Autodesk Inventor part; units mm, degrees
(part 2 of 3)
  spline S285 degree 3 poles (-158.7452, 2.7796) (-159.3519, 3.3863) (-159.5334, 4.2987) (-159.205, 5.0914) knots 0 0 0 0 1 1 1 1 construction
  spline S286 degree 3 poles (-159.205, 5.0914) (-158.8767, 5.8841) (-158.1032, 6.4009) (-157.2452, 6.4009) knots 0 0 0 0 1 1 1 1 construction
  arc A68 (-155.1239, 4.2796) -> (-157.2452, 6.4009) centre (-157.2452, 4.2796) ccw construction
  spline S287 degree 3 poles (-145.4719, 23.3296) (-145.4719, 22.4716) (-145.9887, 21.6981) (-146.7814, 21.3698) knots 0 0 0 0 1 1 1 1 construction
  spline S288 degree 3 poles (-146.7814, 21.3698) (-147.5741, 21.0414) (-148.4865, 21.2229) (-149.0932, 21.8296) knots 0 0 0 0 1 1 1 1 construction
  spline S289 degree 3 poles (-149.0932, 21.8296) (-149.6999, 22.4363) (-149.8814, 23.3487) (-149.553, 24.1414) knots 0 0 0 0 1 1 1 1 construction
  spline S290 degree 3 poles (-149.553, 24.1414) (-149.2247, 24.9341) (-148.4512, 25.4509) (-147.5932, 25.4509) knots 0 0 0 0 1 1 1 1 construction
  arc A69 (-145.4719, 23.3296) -> (-147.5932, 25.4509) centre (-147.5932, 23.3296) ccw construction
  spline S291 degree 3 poles (-136.0739, 4.2796) (-136.0739, 3.4216) (-136.5907, 2.6481) (-137.3834, 2.3198) knots 0 0 0 0 1 1 1 1 construction
  spline S292 degree 3 poles (-137.3834, 2.3198) (-138.1761, 1.9914) (-139.0885, 2.1729) (-139.6952, 2.7796) knots 0 0 0 0 1 1 1 1 construction
  spline S293 degree 3 poles (-139.6952, 2.7796) (-140.3019, 3.3863) (-140.4834, 4.2987) (-140.155, 5.0914) knots 0 0 0 0 1 1 1 1 construction
  spline S294 degree 3 poles (-140.155, 5.0914) (-139.8267, 5.8841) (-139.0532, 6.4009) (-138.1952, 6.4009) knots 0 0 0 0 1 1 1 1 construction
  arc A70 (-136.0739, 4.2796) -> (-138.1952, 6.4009) centre (-138.1952, 4.2796) ccw construction
  spline S295 degree 3 poles (-140.6459, -33.8204) (-140.6459, -34.6784) (-141.1627, -35.4519) (-141.9554, -35.7802) knots 0 0 0 0 1 1 1 1 construction
  spline S296 degree 3 poles (-141.9554, -35.7802) (-142.7481, -36.1086) (-143.6605, -35.9271) (-144.2672, -35.3204) knots 0 0 0 0 1 1 1 1 construction
  spline S297 degree 3 poles (-144.2672, -35.3204) (-144.8739, -34.7137) (-145.0554, -33.8013) (-144.727, -33.0086) knots 0 0 0 0 1 1 1 1 construction
  spline S298 degree 3 poles (-144.727, -33.0086) (-144.3987, -32.2159) (-143.6252, -31.6991) (-142.7672, -31.6991) knots 0 0 0 0 1 1 1 1 construction
  arc A71 (-140.6459, -33.8204) -> (-142.7672, -31.6991) centre (-142.7672, -33.8204) ccw construction
  spline S299 degree 3 poles (-131.2479, -14.7704) (-131.2479, -15.6284) (-131.7647, -16.4019) (-132.5574, -16.7302) knots 0 0 0 0 1 1 1 1 construction
  spline S300 degree 3 poles (-132.5574, -16.7302) (-133.3501, -17.0586) (-134.2625, -16.8771) (-134.8692, -16.2704) knots 0 0 0 0 1 1 1 1 construction
  spline S301 degree 3 poles (-134.8692, -16.2704) (-135.4759, -15.6637) (-135.6574, -14.7513) (-135.329, -13.9586) knots 0 0 0 0 1 1 1 1 construction
  spline S302 degree 3 poles (-135.329, -13.9586) (-135.0007, -13.1659) (-134.2272, -12.6491) (-133.3692, -12.6491) knots 0 0 0 0 1 1 1 1 construction
  arc A72 (-131.2479, -14.7704) -> (-133.3692, -12.6491) centre (-133.3692, -14.7704) ccw construction
  spline S303 degree 3 poles (-121.5959, -33.8204) (-121.5959, -34.6784) (-122.1127, -35.4519) (-122.9054, -35.7802) knots 0 0 0 0 1 1 1 1 construction
  spline S304 degree 3 poles (-122.9054, -35.7802) (-123.6981, -36.1086) (-124.6105, -35.9271) (-125.2172, -35.3204) knots 0 0 0 0 1 1 1 1 construction
  spline S305 degree 3 poles (-125.2172, -35.3204) (-125.8239, -34.7137) (-126.0054, -33.8013) (-125.677, -33.0086) knots 0 0 0 0 1 1 1 1 construction
  spline S306 degree 3 poles (-125.677, -33.0086) (-125.3487, -32.2159) (-124.5752, -31.6991) (-123.7172, -31.6991) knots 0 0 0 0 1 1 1 1 construction
  arc A73 (-121.5959, -33.8204) -> (-123.7172, -31.6991) centre (-123.7172, -33.8204) ccw construction
  arc A74 (-102.5459, -33.8204) -> (-104.6672, -31.6991) centre (-104.6672, -33.8204) ccw construction
  spline S307 degree 3 poles (-102.5459, -33.8204) (-102.5459, -34.6784) (-103.0627, -35.4519) (-103.8554, -35.7802) knots 0 0 0 0 1 1 1 1 construction
  spline S308 degree 3 poles (-103.8554, -35.7802) (-104.6481, -36.1086) (-105.5605, -35.9271) (-106.1672, -35.3204) knots 0 0 0 0 1 1 1 1 construction
  spline S309 degree 3 poles (-106.1672, -35.3204) (-106.7739, -34.7137) (-106.9554, -33.8013) (-106.627, -33.0086) knots 0 0 0 0 1 1 1 1 construction
  spline S310 degree 3 poles (-106.627, -33.0086) (-106.2987, -32.2159) (-105.5252, -31.6991) (-104.6672, -31.6991) knots 0 0 0 0 1 1 1 1 construction
  spline S311 degree 3 poles (-112.1979, -14.7704) (-112.1979, -15.6284) (-112.7147, -16.4019) (-113.5074, -16.7302) knots 0 0 0 0 1 1 1 1 construction
  spline S312 degree 3 poles (-113.5074, -16.7302) (-114.3001, -17.0586) (-115.2125, -16.8771) (-115.8192, -16.2704) knots 0 0 0 0 1 1 1 1 construction
  spline S313 degree 3 poles (-115.8192, -16.2704) (-116.4259, -15.6637) (-116.6074, -14.7513) (-116.279, -13.9586) knots 0 0 0 0 1 1 1 1 construction
  spline S314 degree 3 poles (-116.279, -13.9586) (-115.9507, -13.1659) (-115.1772, -12.6491) (-114.3192, -12.6491) knots 0 0 0 0 1 1 1 1 construction
  arc A75 (-112.1979, -14.7704) -> (-114.3192, -12.6491) centre (-114.3192, -14.7704) ccw construction
  line L28 (-145.8754, -43.9454) -> (-139.8754, -43.9454) construction
  line L29 (-139.8754, -43.9454) -> (-139.8754, -58.9454) construction
  line L30 (-139.8754, -58.9454) -> (-145.8754, -58.9454) construction
  line L31 (-145.8754, -58.9454) -> (-145.8754, -43.9454) construction
  spline S315 degree 3 poles (-134.5894, 49.9986) (-135.3821, 49.6702) (-136.2945, 49.8517) (-136.9012, 50.4584) knots 0 0 0 0 1 1 1 1 construction
  spline S316 degree 3 poles (-136.9012, 50.4584) (-137.5079, 51.0651) (-137.6894, 51.9775) (-137.361, 52.7702) knots 0 0 0 0 1 1 1 1 construction
  spline S317 degree 3 poles (-137.361, 52.7702) (-137.0327, 53.5629) (-136.2592, 54.0797) (-135.4012, 54.0797) knots 0 0 0 0 1 1 1 1 construction
  arc A76 (-133.2799, 51.9584) -> (-135.4012, 54.0797) centre (-135.4012, 51.9584) ccw construction
  spline S318 degree 3 poles (-133.2799, 51.9584) (-133.2799, 51.1004) (-133.7967, 50.3269) (-134.5894, 49.9986) knots 0 0 0 0 1 1 1 1 construction
  spline S319 degree 3 poles (-113.0252, 50.4864) (-113.6319, 51.0931) (-113.8134, 52.0055) (-113.485, 52.7982) knots 0 0 0 0 1 1 1 1 construction
  spline S320 degree 3 poles (-113.485, 52.7982) (-113.1567, 53.5909) (-112.3832, 54.1077) (-111.5252, 54.1077) knots 0 0 0 0 1 1 1 1 construction
  arc A77 (-109.4039, 51.9864) -> (-111.5252, 54.1077) centre (-111.5252, 51.9864) ccw construction
  spline S321 degree 3 poles (-109.4039, 51.9864) (-109.4039, 51.1284) (-109.9207, 50.3549) (-110.7134, 50.0266) knots 0 0 0 0 1 1 1 1 construction
  spline S322 degree 3 poles (-110.7134, 50.0266) (-111.5061, 49.6982) (-112.4185, 49.8797) (-113.0252, 50.4864) knots 0 0 0 0 1 1 1 1 construction
  arc A78 (-108.25, 37.6384) -> (-110, 39.3884) centre (-110, 37.6384) ccw construction
  spline S323 degree 3 poles (-108.25, 37.6384) (-108.25, 36.9306) (-108.6764, 36.2925) (-109.3303, 36.0216) knots 0 0 0 0 1 1 1 1 construction
  spline S324 degree 3 poles (-109.3303, 36.0216) (-109.9842, 35.7507) (-110.7369, 35.9005) (-111.2374, 36.401) knots 0 0 0 0 1 1 1 1 construction
  spline S325 degree 3 poles (-111.2374, 36.401) (-111.7379, 36.9015) (-111.8877, 37.6542) (-111.6168, 38.3081) knots 0 0 0 0 1 1 1 1 construction
  spline S326 degree 3 poles (-111.6168, 38.3081) (-111.3459, 38.962) (-110.7078, 39.3884) (-110, 39.3884) knots 0 0 0 0 1 1 1 1 construction
  arc A79 (-117.0239, 4.2796) -> (-119.1452, 6.4009) centre (-119.1452, 4.2796) ccw construction
  spline S327 degree 3 poles (-117.0239, 4.2796) (-117.0239, 3.4216) (-117.5407, 2.6481) (-118.3334, 2.3198) knots 0 0 0 0 1 1 1 1 construction
  spline S328 degree 3 poles (-118.3334, 2.3198) (-119.1261, 1.9914) (-120.0385, 2.1729) (-120.6452, 2.7796) knots 0 0 0 0 1 1 1 1 construction
  spline S329 degree 3 poles (-120.6452, 2.7796) (-121.2519, 3.3863) (-121.4334, 4.2987) (-121.105, 5.0914) knots 0 0 0 0 1 1 1 1 construction
  spline S330 degree 3 poles (-121.105, 5.0914) (-120.7767, 5.8841) (-120.0032, 6.4009) (-119.1452, 6.4009) knots 0 0 0 0 1 1 1 1 construction
  arc A80 (-107.3719, 23.3296) -> (-109.4932, 25.4509) centre (-109.4932, 23.3296) ccw construction
  spline S331 degree 3 poles (-107.3719, 23.3296) (-107.3719, 22.4716) (-107.8887, 21.6981) (-108.6814, 21.3698) knots 0 0 0 0 1 1 1 1 construction
  spline S332 degree 3 poles (-108.6814, 21.3698) (-109.4741, 21.0414) (-110.3865, 21.2229) (-110.9932, 21.8296) knots 0 0 0 0 1 1 1 1 construction
  spline S333 degree 3 poles (-110.9932, 21.8296) (-111.5999, 22.4363) (-111.7814, 23.3487) (-111.453, 24.1414) knots 0 0 0 0 1 1 1 1 construction
  spline S334 degree 3 poles (-111.453, 24.1414) (-111.1247, 24.9341) (-110.3512, 25.4509) (-109.4932, 25.4509) knots 0 0 0 0 1 1 1 1 construction
  arc A81 (-126.4219, 23.3296) -> (-128.5432, 25.4509) centre (-128.5432, 23.3296) ccw construction
  spline S335 degree 3 poles (-126.4219, 23.3296) (-126.4219, 22.158) (-127.3716, 21.2083) (-128.5432, 21.2083) knots 0 0 0 0 1 1 1 1 construction
  spline S336 degree 3 poles (-128.5432, 21.2083) (-129.7148, 21.2083) (-130.6645, 22.158) (-130.6645, 23.3296) knots 0 0 0 0 1 1 1 1 construction
  spline S337 degree 3 poles (-130.6645, 23.3296) (-130.6645, 24.5012) (-129.7148, 25.4509) (-128.5432, 25.4509) knots 0 0 0 0 1 1 1 1 construction
  arc A82 (-97.9739, 4.2008) -> (-100.0952, 6.3221) centre (-100.0952, 4.2008) ccw construction
  spline S338 degree 3 poles (-97.9739, 4.2008) (-97.9739, 3.3428) (-98.4907, 2.5693) (-99.2834, 2.241) knots 0 0 0 0 1 1 1 1 construction
  spline S339 degree 3 poles (-99.2834, 2.241) (-100.0761, 1.9126) (-100.9885, 2.0941) (-101.5952, 2.7008) knots 0 0 0 0 1 1 1 1 construction
  spline S340 degree 3 poles (-101.5952, 2.7008) (-102.2019, 3.3075) (-102.3834, 4.2199) (-102.055, 5.0126) knots 0 0 0 0 1 1 1 1 construction
  spline S341 degree 3 poles (-102.055, 5.0126) (-101.7267, 5.8053) (-100.9532, 6.3221) (-100.0952, 6.3221) knots 0 0 0 0 1 1 1 1 construction
  spline S342 degree 3 poles (-108.25, -57.5) (-108.25, -58.2078) (-108.6764, -58.8459) (-109.3303, -59.1168) knots 0 0 0 0 1 1 1 1 construction
  spline S343 degree 3 poles (-109.3303, -59.1168) (-109.9842, -59.3877) (-110.7369, -59.2379) (-111.2374, -58.7374) knots 0 0 0 0 1 1 1 1 construction
  spline S344 degree 3 poles (-111.2374, -58.7374) (-111.7379, -58.2369) (-111.8877, -57.4842) (-111.6168, -56.8303) knots 0 0 0 0 1 1 1 1 construction
  spline S345 degree 3 poles (-111.6168, -56.8303) (-111.3459, -56.1764) (-110.7078, -55.75) (-110, -55.75) knots 0 0 0 0 1 1 1 1 construction
  arc A83 (-108.25, -57.5) -> (-110, -55.75) centre (-110, -57.5) ccw construction
  spline S346 degree 3 poles (-93.1479, -14.7704) (-93.1479, -15.6284) (-93.6647, -16.4019) (-94.4574, -16.7302) knots 0 0 0 0 1 1 1 1 construction
  spline S347 degree 3 poles (-94.4574, -16.7302) (-95.2501, -17.0586) (-96.1625, -16.8771) (-96.7692, -16.2704) knots 0 0 0 0 1 1 1 1 construction
  spline S348 degree 3 poles (-96.7692, -16.2704) (-97.3759, -15.6637) (-97.5574, -14.7513) (-97.229, -13.9586) knots 0 0 0 0 1 1 1 1 construction
  spline S349 degree 3 poles (-97.229, -13.9586) (-96.9007, -13.1659) (-96.1272, -12.6491) (-95.2692, -12.6491) knots 0 0 0 0 1 1 1 1 construction
  spline S350 degree 3 poles (-95.2692, -12.6491) (-94.0976, -12.6491) (-93.1479, -13.5988) (-93.1479, -14.7704) knots 0 0 0 0 1 1 1 1 construction
  spline S351 degree 3 poles (-83.4959, -33.8204) (-83.4959, -34.6784) (-84.0127, -35.4519) (-84.8054, -35.7802) knots 0 0 0 0 1 1 1 1 construction
  spline S352 degree 3 poles (-84.8054, -35.7802) (-85.5981, -36.1086) (-86.5105, -35.9271) (-87.1172, -35.3204) knots 0 0 0 0 1 1 1 1 construction
  spline S353 degree 3 poles (-87.1172, -35.3204) (-87.7239, -34.7137) (-87.9054, -33.8013) (-87.577, -33.0086) knots 0 0 0 0 1 1 1 1 construction
  spline S354 degree 3 poles (-87.577, -33.0086) (-87.2487, -32.2159) (-86.4752, -31.6991) (-85.6172, -31.6991) knots 0 0 0 0 1 1 1 1 construction
  spline S355 degree 3 poles (-85.6172, -31.6991) (-84.4456, -31.6991) (-83.4959, -32.6488) (-83.4959, -33.8204) knots 0 0 0 0 1 1 1 1 construction
  spline S356 degree 3 poles (-89.1492, 50.4864) (-89.7559, 51.0931) (-89.9374, 52.0055) (-89.609, 52.7982) knots 0 0 0 0 1 1 1 1 construction
  spline S357 degree 3 poles (-89.609, 52.7982) (-89.2807, 53.5909) (-88.5072, 54.1077) (-87.6492, 54.1077) knots 0 0 0 0 1 1 1 1 construction
  arc A84 (-85.5279, 51.9864) -> (-87.6492, 54.1077) centre (-87.6492, 51.9864) ccw construction
  spline S358 degree 3 poles (-85.5279, 51.9864) (-85.5279, 51.1284) (-86.0447, 50.3549) (-86.8374, 50.0266) knots 0 0 0 0 1 1 1 1 construction
  spline S359 degree 3 poles (-86.8374, 50.0266) (-87.6301, 49.6982) (-88.5425, 49.8797) (-89.1492, 50.4864) knots 0 0 0 0 1 1 1 1 construction
  spline S360 degree 3 poles (-56.6432, 50.4864) (-57.2499, 51.0931) (-57.4314, 52.0055) (-57.103, 52.7982) knots 0 0 0 0 1 1 1 1 construction
  spline S361 degree 3 poles (-57.103, 52.7982) (-56.7747, 53.5909) (-56.0012, 54.1077) (-55.1432, 54.1077) knots 0 0 0 0 1 1 1 1 construction
  arc A85 (-53.0219, 51.9864) -> (-55.1432, 54.1077) centre (-55.1432, 51.9864) ccw construction
  spline S362 degree 3 poles (-53.0219, 51.9864) (-53.0219, 51.1284) (-53.5387, 50.3549) (-54.3314, 50.0266) knots 0 0 0 0 1 1 1 1 construction
  spline S363 degree 3 poles (-54.3314, 50.0266) (-55.1241, 49.6982) (-56.0365, 49.8797) (-56.6432, 50.4864) knots 0 0 0 0 1 1 1 1 construction
  spline S364 degree 3 poles (-72.8932, 21.8296) (-73.4999, 22.4363) (-73.6814, 23.3487) (-73.353, 24.1414) knots 0 0 0 0 1 1 1 1 construction
  spline S365 degree 3 poles (-73.353, 24.1414) (-73.0247, 24.9341) (-72.2512, 25.4509) (-71.3932, 25.4509) knots 0 0 0 0 1 1 1 1 construction
  arc A86 (-69.2719, 23.3296) -> (-71.3932, 25.4509) centre (-71.3932, 23.3296) ccw construction
  spline S366 degree 3 poles (-69.2719, 23.3296) (-69.2719, 22.4716) (-69.7887, 21.6981) (-70.5814, 21.3698) knots 0 0 0 0 1 1 1 1 construction
  spline S367 degree 3 poles (-70.5814, 21.3698) (-71.3741, 21.0414) (-72.2865, 21.2229) (-72.8932, 21.8296) knots 0 0 0 0 1 1 1 1 construction
  spline S368 degree 3 poles (-53.8432, 21.8296) (-54.4499, 22.4363) (-54.6314, 23.3487) (-54.303, 24.1414) knots 0 0 0 0 1 1 1 1 construction
  spline S369 degree 3 poles (-54.303, 24.1414) (-53.9747, 24.9341) (-53.2012, 25.4509) (-52.3432, 25.4509) knots 0 0 0 0 1 1 1 1 construction
  arc A87 (-50.2219, 23.3296) -> (-52.3432, 25.4509) centre (-52.3432, 23.3296) ccw construction
  spline S370 degree 3 poles (-50.2219, 23.3296) (-50.2219, 22.4716) (-50.7387, 21.6981) (-51.5314, 21.3698) knots 0 0 0 0 1 1 1 1 construction
  spline S371 degree 3 poles (-51.5314, 21.3698) (-52.3241, 21.0414) (-53.2365, 21.2229) (-53.8432, 21.8296) knots 0 0 0 0 1 1 1 1 construction
  spline S372 degree 3 poles (-88.3219, 23.3296) (-88.3219, 22.4716) (-88.8387, 21.6981) (-89.6314, 21.3698) knots 0 0 0 0 1 1 1 1 construction
  spline S373 degree 3 poles (-89.6314, 21.3698) (-90.4241, 21.0414) (-91.3365, 21.2229) (-91.9432, 21.8296) knots 0 0 0 0 1 1 1 1 construction
  spline S374 degree 3 poles (-91.9432, 21.8296) (-92.5499, 22.4363) (-92.7314, 23.3487) (-92.403, 24.1414) knots 0 0 0 0 1 1 1 1 construction
  spline S375 degree 3 poles (-92.403, 24.1414) (-92.0747, 24.9341) (-91.3012, 25.4509) (-90.4432, 25.4509) knots 0 0 0 0 1 1 1 1 construction
  spline S376 degree 3 poles (-90.4432, 25.4509) (-89.2716, 25.4509) (-88.3219, 24.5012) (-88.3219, 23.3296) knots 0 0 0 0 1 1 1 1 construction
  spline S377 degree 3 poles (-59.129, -13.9586) (-58.8007, -13.1659) (-58.0272, -12.6491) (-57.1692, -12.6491) knots 0 0 0 0 1 1 1 1 construction
  arc A88 (-55.0479, -14.7704) -> (-57.1692, -12.6491) centre (-57.1692, -14.7704) ccw construction
  spline S378 degree 3 poles (-55.0479, -14.7704) (-55.0479, -15.6284) (-55.5647, -16.4019) (-56.3574, -16.7302) knots 0 0 0 0 1 1 1 1 construction
  spline S379 degree 3 poles (-56.3574, -16.7302) (-57.1501, -17.0586) (-58.0625, -16.8771) (-58.6692, -16.2704) knots 0 0 0 0 1 1 1 1 construction
  spline S380 degree 3 poles (-58.6692, -16.2704) (-59.2759, -15.6637) (-59.4574, -14.7513) (-59.129, -13.9586) knots 0 0 0 0 1 1 1 1 construction
  spline S381 degree 3 poles (-68.527, -33.0086) (-68.1987, -32.2159) (-67.4252, -31.6991) (-66.5672, -31.6991) knots 0 0 0 0 1 1 1 1 construction
  arc A89 (-64.4459, -33.8204) -> (-66.5672, -31.6991) centre (-66.5672, -33.8204) ccw construction
  spline S382 degree 3 poles (-64.4459, -33.8204) (-64.4459, -34.6784) (-64.9627, -35.4519) (-65.7554, -35.7802) knots 0 0 0 0 1 1 1 1 construction
  spline S383 degree 3 poles (-65.7554, -35.7802) (-66.5481, -36.1086) (-67.4605, -35.9271) (-68.0672, -35.3204) knots 0 0 0 0 1 1 1 1 construction
  spline S384 degree 3 poles (-68.0672, -35.3204) (-68.6739, -34.7137) (-68.8554, -33.8013) (-68.527, -33.0086) knots 0 0 0 0 1 1 1 1 construction
  spline S385 degree 3 poles (-78.179, -13.9586) (-77.8507, -13.1659) (-77.0772, -12.6491) (-76.2192, -12.6491) knots 0 0 0 0 1 1 1 1 construction
  arc A90 (-74.0979, -14.7704) -> (-76.2192, -12.6491) centre (-76.2192, -14.7704) ccw construction
  spline S386 degree 3 poles (-74.0979, -14.7704) (-74.0979, -15.6284) (-74.6147, -16.4019) (-75.4074, -16.7302) knots 0 0 0 0 1 1 1 1 construction
  spline S387 degree 3 poles (-75.4074, -16.7302) (-76.2001, -17.0586) (-77.1125, -16.8771) (-77.7192, -16.2704) knots 0 0 0 0 1 1 1 1 construction
  spline S388 degree 3 poles (-77.7192, -16.2704) (-78.3259, -15.6637) (-78.5074, -14.7513) (-78.179, -13.9586) knots 0 0 0 0 1 1 1 1 construction
  arc A91 (-45.3959, -33.8204) -> (-47.5172, -31.6991) centre (-47.5172, -33.8204) ccw construction
  spline S389 degree 3 poles (-45.3959, -33.8204) (-45.3959, -34.6784) (-45.9127, -35.4519) (-46.7054, -35.7802) knots 0 0 0 0 1 1 1 1 construction
  spline S390 degree 3 poles (-46.7054, -35.7802) (-47.4981, -36.1086) (-48.4105, -35.9271) (-49.0172, -35.3204) knots 0 0 0 0 1 1 1 1 construction
  spline S391 degree 3 poles (-49.0172, -35.3204) (-49.6239, -34.7137) (-49.8054, -33.8013) (-49.477, -33.0086) knots 0 0 0 0 1 1 1 1 construction
  spline S392 degree 3 poles (-49.477, -33.0086) (-49.1487, -32.2159) (-48.3752, -31.6991) (-47.5172, -31.6991) knots 0 0 0 0 1 1 1 1 construction
  arc A92 (-74.6059, -52.8704) -> (-76.7272, -50.7491) centre (-76.7272, -52.8704) ccw construction
  spline S393 degree 3 poles (-74.6059, -52.8704) (-74.6059, -53.7284) (-75.1227, -54.5019) (-75.9154, -54.8302) knots 0 0 0 0 1 1 1 1 construction
  spline S394 degree 3 poles (-75.9154, -54.8302) (-76.7081, -55.1586) (-77.6205, -54.9771) (-78.2272, -54.3704) knots 0 0 0 0 1 1 1 1 construction
  spline S395 degree 3 poles (-78.2272, -54.3704) (-78.8339, -53.7637) (-79.0154, -52.8513) (-78.687, -52.0586) knots 0 0 0 0 1 1 1 1 construction
  spline S396 degree 3 poles (-78.687, -52.0586) (-78.3587, -51.2659) (-77.5852, -50.7491) (-76.7272, -50.7491) knots 0 0 0 0 1 1 1 1 construction
  arc A93 (-59.8739, 4.2796) -> (-61.9952, 6.4009) centre (-61.9952, 4.2796) ccw construction
  spline S397 degree 3 poles (-59.8739, 4.2796) (-59.8739, 3.4216) (-60.3907, 2.6481) (-61.1834, 2.3198) knots 0 0 0 0 1 1 1 1 construction
  spline S398 degree 3 poles (-61.1834, 2.3198) (-61.9761, 1.9914) (-62.8885, 2.1729) (-63.4952, 2.7796) knots 0 0 0 0 1 1 1 1 construction
  spline S399 degree 3 poles (-63.4952, 2.7796) (-64.1019, 3.3863) (-64.2834, 4.2987) (-63.955, 5.0914) knots 0 0 0 0 1 1 1 1 construction
  spline S400 degree 3 poles (-63.955, 5.0914) (-63.6267, 5.8841) (-62.8532, 6.4009) (-61.9952, 6.4009) knots 0 0 0 0 1 1 1 1 construction
  arc A94 (-78.9239, 4.2796) -> (-81.0452, 6.4009) centre (-81.0452, 4.2796) ccw construction
  spline S401 degree 3 poles (-78.9239, 4.2796) (-78.9239, 3.4216) (-79.4407, 2.6481) (-80.2334, 2.3198) knots 0 0 0 0 1 1 1 1 construction
  spline S402 degree 3 poles (-80.2334, 2.3198) (-81.0261, 1.9914) (-81.9385, 2.1729) (-82.5452, 2.7796) knots 0 0 0 0 1 1 1 1 construction
  spline S403 degree 3 poles (-82.5452, 2.7796) (-83.1519, 3.3863) (-83.3334, 4.2987) (-83.005, 5.0914) knots 0 0 0 0 1 1 1 1 construction
  spline S404 degree 3 poles (-83.005, 5.0914) (-82.6767, 5.8841) (-81.9032, 6.4009) (-81.0452, 6.4009) knots 0 0 0 0 1 1 1 1 construction
  arc A95 (-40.8239, 4.2796) -> (-42.9452, 6.4009) centre (-42.9452, 4.2796) ccw construction
  spline S405 degree 3 poles (-40.8239, 4.2796) (-40.8239, 3.4216) (-41.3407, 2.6481) (-42.1334, 2.3198) knots 0 0 0 0 1 1 1 1 construction
  spline S406 degree 3 poles (-42.1334, 2.3198) (-42.9261, 1.9914) (-43.8385, 2.1729) (-44.4452, 2.7796) knots 0 0 0 0 1 1 1 1 construction
  spline S407 degree 3 poles (-44.4452, 2.7796) (-45.0519, 3.3863) (-45.2334, 4.2987) (-44.905, 5.0914) knots 0 0 0 0 1 1 1 1 construction
  spline S408 degree 3 poles (-44.905, 5.0914) (-44.5767, 5.8841) (-43.8032, 6.4009) (-42.9452, 6.4009) knots 0 0 0 0 1 1 1 1 construction
  spline S409 degree 3 poles (219.7443, 55.7135) (220.682, 54.7759) (221.2088, 53.5041) (221.2088, 52.178) knots 0 0 0 0 1 1 1 1 construction
  spline S410 degree 3 poles (221.2088, 52.178) (221.2088, 50.1557) (219.9906, 48.3325) (218.1222, 47.5586) knots 0 0 0 0 1 1 1 1 construction
  spline S411 degree 3 poles (218.1222, 47.5586) (216.2538, 46.7847) (214.1033, 47.2125) (212.6733, 48.6425) knots 0 0 0 0 1 1 1 1 construction
  spline S412 degree 3 poles (212.6733, 48.6425) (211.2433, 50.0725) (210.8155, 52.223) (211.5894, 54.0914) knots 0 0 0 0 1 1 1 1 construction
  spline S413 degree 3 poles (211.5894, 54.0914) (212.3633, 55.9598) (214.1865, 57.178) (216.2088, 57.178) knots 0 0 0 0 1 1 1 1 construction
  spline S414 degree 3 poles (216.2088, 57.178) (217.5349, 57.178) (218.8067, 56.6512) (219.7443, 55.7135) knots 0 0 0 0 1 1 1 1 construction
  line L32 (204.7088, -52.274) -> (219.7088, -52.274) construction
  line L33 (219.7088, -52.274) -> (219.7088, -58.274) construction
  line L34 (219.7088, -58.274) -> (204.7088, -58.274) construction
  line L35 (204.7088, -58.274) -> (204.7088, -52.274) construction
  spline S415 degree 3 poles (218.3832, 38.3081) (218.6541, 38.962) (219.2922, 39.3884) (220, 39.3884) knots 0 0 0 0 1 1 1 1 construction
  arc A96 (221.75, 37.6384) -> (220, 39.3884) centre (220, 37.6384) ccw construction
  spline S416 degree 3 poles (221.75, 37.6384) (221.75, 36.9306) (221.3236, 36.2925) (220.6697, 36.0216) knots 0 0 0 0 1 1 1 1 construction
  spline S417 degree 3 poles (220.6697, 36.0216) (220.0158, 35.7507) (219.2631, 35.9005) (218.7626, 36.401) knots 0 0 0 0 1 1 1 1 construction
  spline S418 degree 3 poles (218.7626, 36.401) (218.2621, 36.9015) (218.1123, 37.6542) (218.3832, 38.3081) knots 0 0 0 0 1 1 1 1 construction
  spline S419 degree 3 poles (146.9023, 58.0219) (147.84, 57.0843) (148.3668, 55.8125) (148.3668, 54.4864) knots 0 0 0 0 1 1 1 1 construction
  spline S420 degree 3 poles (148.3668, 54.4864) (148.3668, 52.4641) (147.1486, 50.6409) (145.2802, 49.867) knots 0 0 0 0 1 1 1 1 construction
  spline S421 degree 3 poles (145.2802, 49.867) (143.4118, 49.0931) (141.2613, 49.5209) (139.8313, 50.9509) knots 0 0 0 0 1 1 1 1 construction
  spline S422 degree 3 poles (139.8313, 50.9509) (138.4013, 52.3809) (137.9735, 54.5314) (138.7474, 56.3998) knots 0 0 0 0 1 1 1 1 construction
  spline S423 degree 3 poles (138.7474, 56.3998) (139.5213, 58.2682) (141.3445, 59.4864) (143.3668, 59.4864) knots 0 0 0 0 1 1 1 1 construction
  spline S424 degree 3 poles (143.3668, 59.4864) (144.6929, 59.4864) (145.9647, 58.9596) (146.9023, 58.0219) knots 0 0 0 0 1 1 1 1 construction
  arc A97 (111.75, 37.6384) -> (110, 39.3884) centre (110, 37.6384) ccw construction
  spline S425 degree 3 poles (111.75, 37.6384) (111.75, 36.9306) (111.3236, 36.2925) (110.6697, 36.0216) knots 0 0 0 0 1 1 1 1 construction
  spline S426 degree 3 poles (110.6697, 36.0216) (110.0158, 35.7507) (109.2631, 35.9005) (108.7626, 36.401) knots 0 0 0 0 1 1 1 1 construction
  spline S427 degree 3 poles (108.7626, 36.401) (108.2621, 36.9015) (108.1123, 37.6542) (108.3832, 38.3081) knots 0 0 0 0 1 1 1 1 construction
  spline S428 degree 3 poles (108.3832, 38.3081) (108.6541, 38.962) (109.2922, 39.3884) (110, 39.3884) knots 0 0 0 0 1 1 1 1 construction
  spline S429 degree 3 poles (47.5681, -33.8204) (47.5681, -34.6784) (47.0513, -35.4519) (46.2586, -35.7802) knots 0 0 0 0 1 1 1 1 construction
  spline S430 degree 3 poles (46.2586, -35.7802) (45.4659, -36.1086) (44.5535, -35.9271) (43.9468, -35.3204) knots 0 0 0 0 1 1 1 1 construction
  spline S431 degree 3 poles (43.9468, -35.3204) (43.3401, -34.7137) (43.1586, -33.8013) (43.487, -33.0086) knots 0 0 0 0 1 1 1 1 construction
  spline S432 degree 3 poles (43.487, -33.0086) (43.8153, -32.2159) (44.5888, -31.6991) (45.4468, -31.6991) knots 0 0 0 0 1 1 1 1 construction
  arc A98 (47.5681, -33.8204) -> (45.4468, -31.6991) centre (45.4468, -33.8204) ccw construction
  spline S433 degree 3 poles (218.3832, -23.8303) (218.6541, -23.1764) (219.2922, -22.75) (220, -22.75) knots 0 0 0 0 1 1 1 1 construction
  arc A99 (221.75, -24.5) -> (220, -22.75) centre (220, -24.5) ccw construction
  spline S434 degree 3 poles (221.75, -24.5) (221.75, -25.2078) (221.3236, -25.8459) (220.6697, -26.1168) knots 0 0 0 0 1 1 1 1 construction
  spline S435 degree 3 poles (220.6697, -26.1168) (220.0158, -26.3877) (219.2631, -26.2379) (218.7626, -25.7374) knots 0 0 0 0 1 1 1 1 construction
  spline S436 degree 3 poles (218.7626, -25.7374) (218.2621, -25.2369) (218.1123, -24.4842) (218.3832, -23.8303) knots 0 0 0 0 1 1 1 1 construction
  line L36 (204.7088, -28.274) -> (219.7088, -28.274) construction
  line L37 (219.7088, -28.274) -> (219.7088, -34.274) construction
  line L38 (219.7088, -34.274) -> (204.7088, -34.274) construction
  line L39 (204.7088, -34.274) -> (204.7088, -28.274) construction
  line L40 (151.2108, -58.772) -> (151.2108, -43.772) construction
  line L41 (151.2108, -43.772) -> (157.2108, -43.772) construction
  line L42 (157.2108, -43.772) -> (157.2108, -58.772) construction
  line L43 (157.2108, -58.772) -> (151.2108, -58.772) construction
  line L44 (175.2108, -58.772) -> (175.2108, -43.772) construction
  line L45 (175.2108, -43.772) -> (181.2108, -43.772) construction
  line L46 (181.2108, -43.772) -> (181.2108, -58.772) construction
  line L47 (181.2108, -58.772) -> (175.2108, -58.772) construction
  spline S437 degree 3 poles (191.7443, 55.7135) (192.682, 54.7759) (193.2088, 53.5041) (193.2088, 52.178) knots 0 0 0 0 1 1 1 1 construction
  spline S438 degree 3 poles (193.2088, 52.178) (193.2088, 50.1557) (191.9906, 48.3325) (190.1222, 47.5586) knots 0 0 0 0 1 1 1 1 construction
  spline S439 degree 3 poles (190.1222, 47.5586) (188.2538, 46.7847) (186.1033, 47.2125) (184.6733, 48.6425) knots 0 0 0 0 1 1 1 1 construction
  spline S440 degree 3 poles (184.6733, 48.6425) (183.2433, 50.0725) (182.8155, 52.223) (183.5894, 54.0914) knots 0 0 0 0 1 1 1 1 construction
  spline S441 degree 3 poles (183.5894, 54.0914) (184.3633, 55.9598) (186.1865, 57.178) (188.2088, 57.178) knots 0 0 0 0 1 1 1 1 construction
  spline S442 degree 3 poles (188.2088, 57.178) (189.5349, 57.178) (190.8067, 56.6512) (191.7443, 55.7135) knots 0 0 0 0 1 1 1 1 construction
  line L48 (65.6708, 3.6276) -> (50.6708, 3.6276) construction
  line L49 (50.6708, 3.6276) -> (50.6708, 9.6276) construction
  line L50 (50.6708, 9.6276) -> (65.6708, 9.6276) construction
  line L51 (65.6708, 9.6276) -> (65.6708, 3.6276) construction
  line L52 (-66.3852, 61.3884) -> (51.6148, 61.3884) construction
  line L53 (-66.3852, 42.3884) -> (-66.3852, 61.3884) construction
  line L54 (51.6148, 42.3884) -> (-66.3852, 42.3884) construction
  line L55 (-76.4012, 61.3884) -> (-76.4012, 42.3884) construction
  line L56 (-194.4012, 61.3884) -> (-76.4012, 61.3884) construction
  line L57 (-76.4012, 42.3884) -> (-194.4012, 42.3884) construction
  line L58 (-194.4012, 42.3884) -> (-194.4012, 61.3884) construction
  line L59 (-204.6412, 61.3884) -> (-204.6412, 42.3884) construction
  line L60 (-223.6412, 61.3884) -> (-204.6412, 61.3884) construction
  line L61 (-223.6412, 42.3884) -> (-223.6412, 61.3884) construction
  line L62 (-204.6412, 42.3884) -> (-223.6412, 42.3884) construction
  line L63 (71.4568, 32.8296) -> (-223.6412, 32.8296) construction
  line L64 (-223.6412, 32.8296) -> (-223.6412, -43.3204) construction
  line L65 (-223.6412, -43.3204) -> (-209.6412, -43.3204) construction
  line L66 (-209.6412, -43.3204) -> (-209.6412, -62.3704) construction
  line L67 (-209.6412, -62.3704) -> (57.4568, -62.3704) projected
  line L68 (71.4568, 32.8296) -> (-223.6412, 32.8296) construction
  line L69 (4.4528, 37.558) -> (14.2318, 37.558)
  line L70 (14.2318, 37.558) -> (14.2318, 13.9046)
  line L71 (14.2318, 13.9046) -> (4.4528, 13.9046)
  line L72 (4.4528, 13.9046) -> (4.4528, -5.3455)
  line L73 (4.4528, -5.3455) -> (9.6598, -5.3455)
  line L74 (9.6598, -5.3455) -> (9.6598, -24.1954)
  line L75 (9.6598, -24.1954) -> (0.0048, -24.1954)
  line L76 (0.0048, -24.1954) -> (0.0048, -49.2614)
  line L77 (0.0048, -49.2614) -> (8.4302, -49.2614)
  line L78 (8.4302, -49.2614) -> (8.4302, -62.3704)
  line L79 (4.6528, 61.3884) -> (4.6528, 42.3884) construction
  line L80 (4.6528, 37.758) -> (14.4318, 37.758) construction
  line L81 (14.4318, 32.8296) -> (14.4318, 13.7046) construction
  line L82 (14.4318, 13.7046) -> (4.6528, 13.7046) construction
  line L83 (4.6528, 13.7046) -> (4.6528, -5.1455) construction
  line L84 (4.6528, -5.1455) -> (9.8598, -5.1455) construction
  line L85 (9.8598, -5.1455) -> (9.8598, -24.3954) construction
  line L86 (9.8598, -24.3954) -> (0.2048, -24.3954) construction
  line L87 (0.2048, -24.3954) -> (0.2048, -49.0614) construction
  line L88 (0.2048, -49.0614) -> (8.6302, -49.0614) construction
  line L89 (8.6302, -49.0614) -> (8.6302, -62.3704) construction
  line L90 (4.4528, 61.3884) -> (4.4528, 37.558)
  circle A100 centre (-220, 37.6384) radius 3.25
  circle A101 centre (-220, -24.5) radius 3.25
  circle A102 centre (-110, 37.6384) radius 3.25
  circle A103 centre (0, 37.6384) radius 3.25
  line L91 (-223.6412, 61.3884) -> (-223.6412, -43.3204)
  line L92 (-223.6412, 61.3884) -> (4.4528, 61.3884)
  line L93 (-146.4772, -45.8679) -> (-140.4772, -45.8679)
  line L94 (-140.4772, -45.8679) -> (-140.4772, -58.2679)
  line L95 (-140.4772, -58.2679) -> (-146.4772, -58.2679)
  line L96 (-146.4772, -58.2679) -> (-146.4772, -45.8679)
  line L97 (-12.9772, -45.8679) -> (-6.9772, -45.8679)
  line L98 (-6.9772, -45.8679) -> (-6.9772, -58.2679)
  line L99 (-6.9772, -58.2679) -> (-12.9772, -58.2679)
  line L100 (-12.9772, -58.2679) -> (-12.9772, -45.8679)
  line L101 (-221.1437, 58.8909) -> (-207.1387, 58.8909)
  line L102 (-207.1387, 58.8909) -> (-207.1387, 44.8859)
  line L103 (-207.1387, 44.8859) -> (-221.1437, 44.8859)
  line L104 (-221.1437, 44.8859) -> (-221.1437, 58.8909)
  line L105 (-221.1437, 58.8909) -> (-207.1387, 44.8859) construction
  line L106 (-207.1387, 58.8909) -> (-221.1437, 44.8859) construction
  line L107 (-190.0953, 59.1041) -> (-176.0903, 59.1041)
  line L108 (-176.0903, 59.1041) -> (-176.0903, 45.0991)
  line L109 (-176.0903, 45.0991) -> (-190.0953, 45.0991)
  line L110 (-190.0953, 45.0991) -> (-190.0953, 59.1041)
  line L111 (-190.0953, 59.1041) -> (-176.0903, 45.0991) construction
  line L112 (-176.0903, 59.1041) -> (-190.0953, 45.0991) construction
  line L113 (-166.2797, 58.9889) -> (-152.2747, 58.9889)
  line L114 (-152.2747, 58.9889) -> (-152.2747, 44.9839)
  line L115 (-152.2747, 44.9839) -> (-166.2797, 44.9839)
  line L116 (-166.2797, 44.9839) -> (-166.2797, 58.9889)
  line L117 (-166.2797, 58.9889) -> (-152.2747, 44.9839) construction
  line L118 (-152.2747, 58.9889) -> (-166.2797, 44.9839) construction
  line L119 (-142.4037, 58.9609) -> (-128.3987, 58.9609)
  line L120 (-128.3987, 58.9609) -> (-128.3987, 44.9559)
  line L121 (-128.3987, 44.9559) -> (-142.4037, 44.9559)
  line L122 (-142.4037, 44.9559) -> (-142.4037, 58.9609)
  line L123 (-142.4037, 58.9609) -> (-128.3987, 44.9559) construction
  line L124 (-128.3987, 58.9609) -> (-142.4037, 44.9559) construction
  line L125 (-118.5277, 58.9889) -> (-104.5227, 58.9889)
  line L126 (-104.5227, 58.9889) -> (-104.5227, 44.9839)
  line L127 (-104.5227, 44.9839) -> (-118.5277, 44.9839)
  line L128 (-118.5277, 44.9839) -> (-118.5277, 58.9889)
  line L129 (-118.5277, 58.9889) -> (-104.5227, 44.9839) construction
  line L130 (-104.5227, 58.9889) -> (-118.5277, 44.9839) construction
  line L131 (-94.6517, 58.9889) -> (-80.6467, 58.9889)
  line L132 (-80.6467, 58.9889) -> (-80.6467, 44.9839)
  line L133 (-80.6467, 44.9839) -> (-94.6517, 44.9839)
  line L134 (-94.6517, 44.9839) -> (-94.6517, 58.9889)
  line L135 (-94.6517, 58.9889) -> (-80.6467, 44.9839) construction
  line L136 (-80.6467, 58.9889) -> (-94.6517, 44.9839) construction
  line L137 (-62.1457, 58.9889) -> (-48.1407, 58.9889)
  line L138 (-48.1407, 58.9889) -> (-48.1407, 44.9839)
  line L139 (-48.1407, 44.9839) -> (-62.1457, 44.9839)
  line L140 (-62.1457, 44.9839) -> (-62.1457, 58.9889)
  line L141 (-62.1457, 58.9889) -> (-48.1407, 44.9839) construction
  line L142 (-48.1407, 58.9889) -> (-62.1457, 44.9839) construction
  line L143 (-38.2637, 58.9889) -> (-24.2587, 58.9889)
  line L144 (-24.2587, 58.9889) -> (-24.2587, 44.9839)
  line L145 (-24.2587, 44.9839) -> (-38.2637, 44.9839)
  line L146 (-38.2637, 44.9839) -> (-38.2637, 58.9889)
  line L147 (-38.2637, 58.9889) -> (-24.2587, 44.9839) construction
  line L148 (-24.2587, 58.9889) -> (-38.2637, 44.9839) construction
  line L149 (-14.3877, 58.9889) -> (-0.3827, 58.9889)
  line L150 (-0.3827, 58.9889) -> (-0.3827, 44.9839)
  line L151 (-0.3827, 44.9839) -> (-14.3877, 44.9839)
  line L152 (-14.3877, 44.9839) -> (-14.3877, 58.9889)
  line L153 (-14.3877, 58.9889) -> (-0.3827, 44.9839) construction
  line L154 (-0.3827, 58.9889) -> (-14.3877, 44.9839) construction
  line L155 (-216.4737, 30.3321) -> (-202.4687, 30.3321)
  line L156 (-202.4687, 30.3321) -> (-202.4687, 16.3271)
  line L157 (-202.4687, 16.3271) -> (-216.4737, 16.3271)
  line L158 (-216.4737, 16.3271) -> (-216.4737, 30.3321)
  line L159 (-216.4737, 30.3321) -> (-202.4687, 16.3271) construction
  line L160 (-202.4687, 30.3321) -> (-216.4737, 16.3271) construction
  line L161 (-192.6957, 30.3321) -> (-178.6907, 30.3321)
  line L162 (-178.6907, 30.3321) -> (-178.6907, 16.3271)
  line L163 (-178.6907, 16.3271) -> (-192.6957, 16.3271)
  line L164 (-192.6957, 16.3271) -> (-192.6957, 30.3321)
  line L165 (-192.6957, 30.3321) -> (-178.6907, 16.3271) construction
  line L166 (-178.6907, 30.3321) -> (-192.6957, 16.3271) construction
  line L167 (-154.5957, 30.3321) -> (-140.5907, 30.3321)
  line L168 (-140.5907, 30.3321) -> (-140.5907, 16.3271)
  line L169 (-140.5907, 16.3271) -> (-154.5957, 16.3271)
  line L170 (-154.5957, 16.3271) -> (-154.5957, 30.3321)
  line L171 (-154.5957, 30.3321) -> (-140.5907, 16.3271) construction
  line L172 (-140.5907, 30.3321) -> (-154.5957, 16.3271) construction
  line L173 (-135.5457, 30.3321) -> (-121.5407, 30.3321)
  line L174 (-121.5407, 30.3321) -> (-121.5407, 16.3271)
  line L175 (-121.5407, 16.3271) -> (-135.5457, 16.3271)
  line L176 (-135.5457, 16.3271) -> (-135.5457, 30.3321)
  line L177 (-135.5457, 30.3321) -> (-121.5407, 16.3271) construction
  line L178 (-121.5407, 30.3321) -> (-135.5457, 16.3271) construction
  line L179 (-116.4957, 30.3321) -> (-102.4907, 30.3321)
  line L180 (-102.4907, 30.3321) -> (-102.4907, 16.3271)
  line L181 (-102.4907, 16.3271) -> (-116.4957, 16.3271)
  line L182 (-116.4957, 16.3271) -> (-116.4957, 30.3321)
  line L183 (-116.4957, 30.3321) -> (-102.4907, 16.3271) construction
  line L184 (-102.4907, 30.3321) -> (-116.4957, 16.3271) construction
  line L185 (-97.4457, 30.3321) -> (-83.4407, 30.3321)
  line L186 (-83.4407, 30.3321) -> (-83.4407, 16.3271)
  line L187 (-83.4407, 16.3271) -> (-97.4457, 16.3271)
  line L188 (-97.4457, 16.3271) -> (-97.4457, 30.3321)
  line L189 (-97.4457, 30.3321) -> (-83.4407, 16.3271) construction
  line L190 (-83.4407, 30.3321) -> (-97.4457, 16.3271) construction
  line L191 (-173.6457, 30.3321) -> (-159.6407, 30.3321)
  line L192 (-159.6407, 30.3321) -> (-159.6407, 16.3271)
  line L193 (-159.6407, 16.3271) -> (-173.6457, 16.3271)
  line L194 (-173.6457, 16.3271) -> (-173.6457, 30.3321)
  line L195 (-173.6457, 30.3321) -> (-159.6407, 16.3271) construction
  line L196 (-159.6407, 30.3321) -> (-173.6457, 16.3271) construction
  line L197 (-78.3957, 30.3321) -> (-64.3907, 30.3321)
  line L198 (-64.3907, 30.3321) -> (-64.3907, 16.3271)
  line L199 (-64.3907, 16.3271) -> (-78.3957, 16.3271)
  line L200 (-78.3957, 16.3271) -> (-78.3957, 30.3321)
  line L201 (-78.3957, 30.3321) -> (-64.3907, 16.3271) construction
  line L202 (-64.3907, 30.3321) -> (-78.3957, 16.3271) construction
  line L203 (-59.3457, 30.3321) -> (-45.3407, 30.3321)
  line L204 (-45.3407, 30.3321) -> (-45.3407, 16.3271)
  line L205 (-45.3407, 16.3271) -> (-59.3457, 16.3271)
  line L206 (-59.3457, 16.3271) -> (-59.3457, 30.3321)
  line L207 (-59.3457, 30.3321) -> (-45.3407, 16.3271) construction
  line L208 (-45.3407, 30.3321) -> (-59.3457, 16.3271) construction
  line L209 (-40.2957, 30.3321) -> (-26.2907, 30.3321)
  line L210 (-26.2907, 30.3321) -> (-26.2907, 16.3271)
  line L211 (-26.2907, 16.3271) -> (-40.2957, 16.3271)
  line L212 (-40.2957, 16.3271) -> (-40.2957, 30.3321)
  line L213 (-40.2957, 30.3321) -> (-26.2907, 16.3271) construction
  line L214 (-26.2907, 30.3321) -> (-40.2957, 16.3271) construction
  line L215 (-21.2457, 30.3321) -> (-7.2407, 30.3321)
  line L216 (-7.2407, 30.3321) -> (-7.2407, 16.3271)
  line L217 (-7.2407, 16.3271) -> (-21.2457, 16.3271)
  line L218 (-21.2457, 16.3271) -> (-21.2457, 30.3321)
  line L219 (-21.2457, 30.3321) -> (-7.2407, 16.3271) construction
  line L220 (-7.2407, 30.3321) -> (-21.2457, 16.3271) construction
  line L221 (-2.1957, 30.3321) -> (11.8093, 30.3321)
  line L222 (11.8093, 30.3321) -> (11.8093, 16.3271)
  line L223 (11.8093, 16.3271) -> (-2.1957, 16.3271)
  line L224 (-2.1957, 16.3271) -> (-2.1957, 30.3321)
  line L225 (-2.1957, 30.3321) -> (11.8093, 16.3271) construction
  line L226 (11.8093, 30.3321) -> (-2.1957, 16.3271) construction
  line L227 (-11.8477, 11.2821) -> (2.1573, 11.2821)
  line L228 (2.1573, 11.2821) -> (2.1573, -2.7229)
  line L229 (2.1573, -2.7229) -> (-11.8477, -2.7229)
  line L230 (-11.8477, -2.7229) -> (-11.8477, 11.2821)
  line L231 (-11.8477, 11.2821) -> (2.1573, -2.7229) construction
  line L232 (2.1573, 11.2821) -> (-11.8477, -2.7229) construction
  line L233 (-30.8977, 11.2821) -> (-16.8927, 11.2821)
  line L234 (-16.8927, 11.2821) -> (-16.8927, -2.7229)
  line L235 (-16.8927, -2.7229) -> (-30.8977, -2.7229)
  line L236 (-30.8977, -2.7229) -> (-30.8977, 11.2821)
  line L237 (-30.8977, 11.2821) -> (-16.8927, -2.7229) construction
  line L238 (-16.8927, 11.2821) -> (-30.8977, -2.7229) construction
  line L239 (-49.9477, 11.2821) -> (-35.9427, 11.2821)
  line L240 (-35.9427, 11.2821) -> (-35.9427, -2.7229)
  line L241 (-35.9427, -2.7229) -> (-49.9477, -2.7229)
  line L242 (-49.9477, -2.7229) -> (-49.9477, 11.2821)
  line L243 (-49.9477, 11.2821) -> (-35.9427, -2.7229) construction
  line L244 (-35.9427, 11.2821) -> (-49.9477, -2.7229) construction
  line L245 (-68.9977, 11.2821) -> (-54.9927, 11.2821)
  line L246 (-54.9927, 11.2821) -> (-54.9927, -2.7229)
  line L247 (-54.9927, -2.7229) -> (-68.9977, -2.7229)
  line L248 (-68.9977, -2.7229) -> (-68.9977, 11.2821)
  line L249 (-68.9977, 11.2821) -> (-54.9927, -2.7229) construction
  line L250 (-54.9927, 11.2821) -> (-68.9977, -2.7229) construction
  line L251 (-88.0477, 11.2821) -> (-74.0427, 11.2821)
  line L252 (-74.0427, 11.2821) -> (-74.0427, -2.7229)
  line L253 (-74.0427, -2.7229) -> (-88.0477, -2.7229)
  line L254 (-88.0477, -2.7229) -> (-88.0477, 11.2821)
  line L255 (-88.0477, 11.2821) -> (-74.0427, -2.7229) construction
  line L256 (-74.0427, 11.2821) -> (-88.0477, -2.7229) construction
  line L257 (-107.0977, 11.2033) -> (-93.0927, 11.2033)
  line L258 (-93.0927, 11.2033) -> (-93.0927, -2.8017)
  line L259 (-93.0927, -2.8017) -> (-107.0977, -2.8017)
  line L260 (-107.0977, -2.8017) -> (-107.0977, 11.2033)
  line L261 (-107.0977, 11.2033) -> (-93.0927, -2.8017) construction
  line L262 (-93.0927, 11.2033) -> (-107.0977, -2.8017) construction
  line L263 (-112.1427, 11.2821) -> (-126.1477, 11.2821)
  line L264 (-126.1477, 11.2821) -> (-126.1477, -2.7229)
  line L265 (-126.1477, -2.7229) -> (-112.1427, -2.7229)
  line L266 (-112.1427, -2.7229) -> (-112.1427, 11.2821)
  line L267 (-112.1427, 11.2821) -> (-126.1477, -2.7229) construction
  line L268 (-126.1477, 11.2821) -> (-112.1427, -2.7229) construction
  line L269 (-145.1977, 11.2821) -> (-131.1927, 11.2821)
  line L270 (-131.1927, 11.2821) -> (-131.1927, -2.7229)
  line L271 (-131.1927, -2.7229) -> (-145.1977, -2.7229)
  line L272 (-145.1977, -2.7229) -> (-145.1977, 11.2821)
  line L273 (-145.1977, 11.2821) -> (-131.1927, -2.7229) construction
  line L274 (-131.1927, 11.2821) -> (-145.1977, -2.7229) construction
  line L275 (-164.2477, 11.2821) -> (-150.2427, 11.2821)
  line L276 (-150.2427, 11.2821) -> (-150.2427, -2.7229)
  line L277 (-150.2427, -2.7229) -> (-164.2477, -2.7229)
  line L278 (-164.2477, -2.7229) -> (-164.2477, 11.2821)
  line L279 (-164.2477, 11.2821) -> (-150.2427, -2.7229) construction
  line L280 (-150.2427, 11.2821) -> (-164.2477, -2.7229) construction
  line L281 (-183.2977, 11.2821) -> (-169.2927, 11.2821)
  line L282 (-169.2927, 11.2821) -> (-169.2927, -2.7229)
  line L283 (-169.2927, -2.7229) -> (-183.2977, -2.7229)
  line L284 (-183.2977, -2.7229) -> (-183.2977, 11.2821)
  line L285 (-183.2977, 11.2821) -> (-169.2927, -2.7229) construction
  line L286 (-169.2927, 11.2821) -> (-183.2977, -2.7229) construction
  line L287 (-211.7457, 11.2821) -> (-197.7407, 11.2821)
  line L288 (-197.7407, 11.2821) -> (-197.7407, -2.7229)
  line L289 (-197.7407, -2.7229) -> (-211.7457, -2.7229)
  line L290 (-211.7457, -2.7229) -> (-211.7457, 11.2821)
  line L291 (-211.7457, 11.2821) -> (-197.7407, -2.7229) construction
  line L292 (-197.7407, 11.2821) -> (-211.7457, -2.7229) construction
  line L293 (-218.8577, -7.7679) -> (-204.8527, -7.7679)
  line L294 (-204.8527, -7.7679) -> (-204.8527, -21.7729)
  line L295 (-204.8527, -21.7729) -> (-218.8577, -21.7729)
  line L296 (-218.8577, -21.7729) -> (-218.8577, -7.7679)
  line L297 (-218.8577, -7.7679) -> (-204.8527, -21.7729) construction
  line L298 (-204.8527, -7.7679) -> (-218.8577, -21.7729) construction
  line L299 (-197.5217, -7.7679) -> (-183.5167, -7.7679)
  line L300 (-183.5167, -7.7679) -> (-183.5167, -21.7729)
  line L301 (-183.5167, -21.7729) -> (-197.5217, -21.7729)
  line L302 (-197.5217, -21.7729) -> (-197.5217, -7.7679)
  line L303 (-197.5217, -7.7679) -> (-183.5167, -21.7729) construction
  line L304 (-183.5167, -7.7679) -> (-197.5217, -21.7729) construction
  line L305 (-178.4717, -7.7679) -> (-164.4667, -7.7679)
  line L306 (-164.4667, -7.7679) -> (-164.4667, -21.7729)
  line L307 (-164.4667, -21.7729) -> (-178.4717, -21.7729)
  line L308 (-178.4717, -21.7729) -> (-178.4717, -7.7679)
  line L309 (-178.4717, -7.7679) -> (-164.4667, -21.7729) construction
  line L310 (-164.4667, -7.7679) -> (-178.4717, -21.7729) construction
  line L311 (-159.4217, -7.7679) -> (-145.4167, -7.7679)
  line L312 (-145.4167, -7.7679) -> (-145.4167, -21.7729)
  line L313 (-145.4167, -21.7729) -> (-159.4217, -21.7729)
  line L314 (-159.4217, -21.7729) -> (-159.4217, -7.7679)
  line L315 (-159.4217, -7.7679) -> (-145.4167, -21.7729) construction
  line L316 (-145.4167, -7.7679) -> (-159.4217, -21.7729) construction
  line L317 (-140.3717, -7.7679) -> (-126.3667, -7.7679)
  line L318 (-126.3667, -7.7679) -> (-126.3667, -21.7729)
  line L319 (-126.3667, -21.7729) -> (-140.3717, -21.7729)
  line L320 (-140.3717, -21.7729) -> (-140.3717, -7.7679)
  line L321 (-140.3717, -7.7679) -> (-126.3667, -21.7729) construction
  line L322 (-126.3667, -7.7679) -> (-140.3717, -21.7729) construction
  line L323 (-121.3217, -7.7679) -> (-107.3167, -7.7679)
  line L324 (-107.3167, -7.7679) -> (-107.3167, -21.7729)
  line L325 (-107.3167, -21.7729) -> (-121.3217, -21.7729)
  line L326 (-121.3217, -21.7729) -> (-121.3217, -7.7679)
  line L327 (-121.3217, -7.7679) -> (-107.3167, -21.7729) construction
  line L328 (-107.3167, -7.7679) -> (-121.3217, -21.7729) construction
  line L329 (-102.2717, -7.7679) -> (-88.2667, -7.7679)
  line L330 (-88.2667, -7.7679) -> (-88.2667, -21.7729)
  line L331 (-88.2667, -21.7729) -> (-102.2717, -21.7729)
  line L332 (-102.2717, -21.7729) -> (-102.2717, -7.7679)
  line L333 (-102.2717, -7.7679) -> (-88.2667, -21.7729) construction
  line L334 (-88.2667, -7.7679) -> (-102.2717, -21.7729) construction
  line L335 (-83.2217, -7.7679) -> (-69.2167, -7.7679)
  line L336 (-69.2167, -7.7679) -> (-69.2167, -21.7729)
  line L337 (-69.2167, -21.7729) -> (-83.2217, -21.7729)
  line L338 (-83.2217, -21.7729) -> (-83.2217, -7.7679)
  line L339 (-83.2217, -7.7679) -> (-69.2167, -21.7729) construction
  line L340 (-69.2167, -7.7679) -> (-83.2217, -21.7729) construction
  line L341 (-64.1717, -7.7679) -> (-50.1667, -7.7679)
  line L342 (-50.1667, -7.7679) -> (-50.1667, -21.7729)
  line L343 (-50.1667, -21.7729) -> (-64.1717, -21.7729)
  line L344 (-64.1717, -21.7729) -> (-64.1717, -7.7679)
  line L345 (-64.1717, -7.7679) -> (-50.1667, -21.7729) construction
  line L346 (-50.1667, -7.7679) -> (-64.1717, -21.7729) construction
  line L347 (-45.1217, -7.7679) -> (-31.1167, -7.7679)
  line L348 (-31.1167, -7.7679) -> (-31.1167, -21.7729)
  line L349 (-31.1167, -21.7729) -> (-45.1217, -21.7729)
  line L350 (-45.1217, -21.7729) -> (-45.1217, -7.7679)
  line L351 (-45.1217, -7.7679) -> (-31.1167, -21.7729) construction
  line L352 (-31.1167, -7.7679) -> (-45.1217, -21.7729) construction
  line L353 (-26.0717, -7.7679) -> (-12.0667, -7.7679)
  line L354 (-12.0667, -7.7679) -> (-12.0667, -21.7729)
  line L355 (-12.0667, -21.7729) -> (-26.0717, -21.7729)
  line L356 (-26.0717, -21.7729) -> (-26.0717, -7.7679)
  line L357 (-26.0717, -7.7679) -> (-12.0667, -21.7729) construction
  line L358 (-12.0667, -7.7679) -> (-26.0717, -21.7729) construction
  line L359 (-6.7677, -7.7679) -> (7.2373, -7.7679)
  line L360 (7.2373, -7.7679) -> (7.2373, -21.7729)
  line L361 (7.2373, -21.7729) -> (-6.7677, -21.7729)
  line L362 (-6.7677, -21.7729) -> (-6.7677, -7.7679)
  line L363 (-6.7677, -7.7679) -> (7.2373, -21.7729) construction
  line L364 (7.2373, -7.7679) -> (-6.7677, -21.7729) construction
  line L365 (-16.4257, -26.8399) -> (-2.4207, -26.8399)
  line L366 (-2.4207, -26.8399) -> (-2.4207, -40.8449)
  line L367 (-2.4207, -40.8449) -> (-16.4257, -40.8449)
  line L368 (-16.4257, -40.8449) -> (-16.4257, -26.8399)
  line L369 (-16.4257, -26.8399) -> (-2.4207, -40.8449) construction
  line L370 (-2.4207, -26.8399) -> (-16.4257, -40.8449) construction
  line L371 (-35.4757, -26.8399) -> (-21.4707, -26.8399)
  line L372 (-21.4707, -26.8399) -> (-21.4707, -40.8449)
  line L373 (-21.4707, -40.8449) -> (-35.4757, -40.8449)
  line L374 (-35.4757, -40.8449) -> (-35.4757, -26.8399)
  line L375 (-35.4757, -26.8399) -> (-21.4707, -40.8449) construction
  line L376 (-21.4707, -26.8399) -> (-35.4757, -40.8449) construction
  line L377 (-54.5197, -26.8179) -> (-40.5147, -26.8179)
  line L378 (-40.5147, -26.8179) -> (-40.5147, -40.8229)
  line L379 (-40.5147, -40.8229) -> (-54.5197, -40.8229)
  line L380 (-54.5197, -40.8229) -> (-54.5197, -26.8179)
  line L381 (-54.5197, -26.8179) -> (-40.5147, -40.8229) construction
  line L382 (-40.5147, -26.8179) -> (-54.5197, -40.8229) construction
  line L383 (-73.5697, -26.8179) -> (-59.5647, -26.8179)
  line L384 (-59.5647, -26.8179) -> (-59.5647, -40.8229)
  line L385 (-59.5647, -40.8229) -> (-73.5697, -40.8229)
  line L386 (-73.5697, -40.8229) -> (-73.5697, -26.8179)
  line L387 (-73.5697, -26.8179) -> (-59.5647, -40.8229) construction
  line L388 (-59.5647, -26.8179) -> (-73.5697, -40.8229) construction
  line L389 (-92.6197, -26.8179) -> (-78.6147, -26.8179)
  line L390 (-78.6147, -26.8179) -> (-78.6147, -40.8229)
  line L391 (-78.6147, -40.8229) -> (-92.6197, -40.8229)
  line L392 (-92.6197, -40.8229) -> (-92.6197, -26.8179)
  line L393 (-92.6197, -26.8179) -> (-78.6147, -40.8229) construction
  line L394 (-78.6147, -26.8179) -> (-92.6197, -40.8229) construction
  line L395 (-111.6697, -26.8179) -> (-97.6647, -26.8179)
  line L396 (-97.6647, -26.8179) -> (-97.6647, -40.8229)
  line L397 (-97.6647, -40.8229) -> (-111.6697, -40.8229)
  line L398 (-111.6697, -40.8229) -> (-111.6697, -26.8179)
  line L399 (-111.6697, -26.8179) -> (-97.6647, -40.8229) construction
  line L400 (-97.6647, -26.8179) -> (-111.6697, -40.8229) construction
  line L401 (-130.7197, -26.8179) -> (-116.7147, -26.8179)
  line L402 (-116.7147, -26.8179) -> (-116.7147, -40.8229)
  line L403 (-116.7147, -40.8229) -> (-130.7197, -40.8229)
  line L404 (-130.7197, -40.8229) -> (-130.7197, -26.8179)
  line L405 (-130.7197, -26.8179) -> (-116.7147, -40.8229) construction
  line L406 (-116.7147, -26.8179) -> (-130.7197, -40.8229) construction
  line L407 (-149.7697, -26.8179) -> (-135.7647, -26.8179)
  line L408 (-135.7647, -26.8179) -> (-135.7647, -40.8229)
  line L409 (-135.7647, -40.8229) -> (-149.7697, -40.8229)
  line L410 (-149.7697, -40.8229) -> (-149.7697, -26.8179)
  line L411 (-149.7697, -26.8179) -> (-135.7647, -40.8229) construction
  line L412 (-135.7647, -26.8179) -> (-149.7697, -40.8229) construction
  line L413 (-168.8197, -26.8179) -> (-154.8147, -26.8179)
  line L414 (-154.8147, -26.8179) -> (-154.8147, -40.8229)